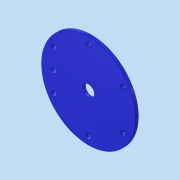
# Autodesk Inventor part: pistonSealingWallFront
Saved by Autodesk Inventor 2017 (Build 210142000, 142)
## iProperties
Created: 2016-11-26
Part Number: pistonSealingWallFront
Material: ABS Plastic
Document SubType Name: Modeling
Designer: techn
Density: 1.06 g/cm^3
Appearance: Blue - Wall Paint - Glossy
Author: techn
Autodesk Inventor part; units mm, degrees
ref_plane "YZ Plane" through (0, 0, 0) normal (1, 0, 0) x (0, 1, 0)
ref_plane "XZ Plane" through (0, 0, 0) normal (0, 1, 0) x (-1, 0, 0)
ref_plane "XY Plane" through (0, 0, 0) normal (0, 0, 1) x (1, 0, 0)
sketch "Sketch1" plane through (0, 0, 0) normal (0, 0, 1) x (1, 0, 0)
  circle A0 centre (0, 0) radius 34.544
  dimension "d0" = 69.088
  constraints: 1 centre point, 1 coincident
  measures "d0" diameter of A0
extrude "Extrusion1" add sketch "Sketch1" along normal blind 2.032
sketch "Sketch2" plane through (0, 0, 2.032) normal (0, 0, 1) x (1, 0, 0)
  line L0 (0, 0) -> (0, 29.21)
  circle A0 centre (0, 29.21) radius 1.8415
  circle A1 centre (-25.2966, 14.605) radius 1.8415
  circle A2 centre (-25.2966, -14.605) radius 1.8415
  circle A3 centre (0, -29.21) radius 1.8415
  circle A4 centre (25.2966, -14.605) radius 1.8415
  circle A5 centre (25.2966, 14.605) radius 1.8415
  dimension "d3" = 29.21
  dimension "d4" = 3.683
  dimension "d7" = 360
  constraints: 6 centre point, 2 end point, 1 coincident, 1 vertical, 13 other
  measures "d3" distance of L0.start L0.end
  measures "d4" diameter of A0
extrude "Extrusion2" cut sketch "Sketch2" against normal blind 2.4765
sketch "Sketch3" plane through (0, 0, 0) normal (0, 0, -1) x (-1, 0, 0)
  line L0 (0, 0) -> (25.4, 0)
  circle A0 centre (25.4, 0) radius 1.8415
  dimension "d11" = 25.4
  dimension "d12" = 3.683
  constraints: 2 end point, 1 centre point, 1 coincident, 1 horizontal
  measures "d11" distance of L0.start L0.end
  measures "d12" diameter of A0
extrude "Extrusion3" cut sketch "Sketch3" against normal blind 2.4765
sketch "Sketch4" plane through (0, 0, 0) normal (0, 0, -1) x (-1, 0, 0)
  circle A0 centre (0, 0) radius 4.318
  dimension "d15" = 8.636
  constraints: 1 centre point, 1 coincident
  measures "d15" diameter of A0
extrude "Extrusion4" cut sketch "Sketch4" against normal blind 2.4765
body "Solid1"
